GearMounts v6 (Autodesk Fusion 360 design; units mm, degrees)
Autodesk Fusion 360 part; units mm, degrees
sketch "Sketch1" plane through (0, 0, 0) normal (0, 1, 0) x (1, 0, 0)
  line L0 (0, 0) -> (122, 0)
  line L1 (122, 0) -> (122, -62)
  line L2 (122, -62) -> (0, -62)
  line L3 (0, -62) -> (0, 0)
  dimension "d1" = 62
  dimension "d2" = 122
  constraint horizontal L0
  constraint vertical L1
  constraint horizontal L2
  constraint vertical L3
  constraint coincident L0.start L3.end
  measures "d1" distance of L0.start
extrude "Extrude1" add sketch "Sketch1" along normal blind 3
sketch "Sketch2" plane through (0, 3, 0) normal (0, 1, 0) x (-1, 0, 0)
  line L0 (0, 62) -> (-122, 62)
  line L1 (-122, 62) -> (-122, 0)
  line L2 (-122, 0) -> (0, 0)
  line L3 (0, 0) -> (0, 62)
  circle A0 centre (-19, 31) radius 5
  circle A1 centre (-63.979, 31) radius 10
  dimension "d5" = 19
  dimension "d6" = 10
  dimension "d7" = 20
  dimension "d8" = 44.979
  measures "d5" distance of L3
  measures "d6" diameter of A0
  measures "d7" diameter of A1
extrude "Extrude2" add sketch "Sketch2" along normal blind 7.05 contours A0 | A1
sketch "Sketch3" plane through (0, 10.05, 0) normal (0, 1, 0) x (-1, 0, 0)
  circle A0 centre (-19, 31) radius 5
  circle A1 centre (-19, 31) radius 1.5
  dimension "d11" = 3
  constraint concentric A0 A1
  measures "d11" diameter of A1
extrude "Extrude3" add sketch "Sketch3" along normal blind 5 contours A1
sketch "Sketch4" plane through (0, 10.05, 0) normal (0, 1, 0) x (-1, 0, 0)
  circle A0 centre (-63.979, 31) radius 10
  circle A1 centre (-63.979, 31) radius 5.1
  dimension "d14" = 10.2
  constraint concentric A0 A1
  measures "d14" diameter of A1
extrude "Extrude4" cut sketch "Sketch4" against normal up to surface (7.05 mm away) contours A1
sketch "Sketch5" plane through (0, 3, 0) normal (0, 1, 0) x (-1, 0, 0)
  circle A0 centre (-63.979, 31) radius 5.1
  circle A1 centre (-63.979, 31) radius 5.1
  line L0 (-53, 21.95) -> (-80, 21.95)
  line L1 (-80, 21.95) -> (-80, 26.95)
  line L2 (-80, 26.95) -> (-53, 26.95)
  line L3 (-53, 26.95) -> (-53, 21.95)
  line L4 (-52, 40.05) -> (-79, 40.05)
  line L5 (-79, 40.05) -> (-79, 35.05)
  line L6 (-79, 35.05) -> (-52, 35.05)
  line L7 (-52, 35.05) -> (-52, 40.05)
  dimension "d17" = 8.1
  dimension "d18" = 5
  dimension "d19" = 5
  dimension "d20" = 4.05
  constraint concentric A0 A1
  constraint horizontal L0
  constraint vertical L1
  constraint horizontal L2
  constraint vertical L3
  constraint horizontal L4
  constraint vertical L5
  constraint horizontal L6
  constraint vertical L7
  measures "d17" distance of L2 L6
extrude "Extrude5" cut sketch "Sketch5" against normal up to surface (3 mm away) contours A0 A1 L2 L6
